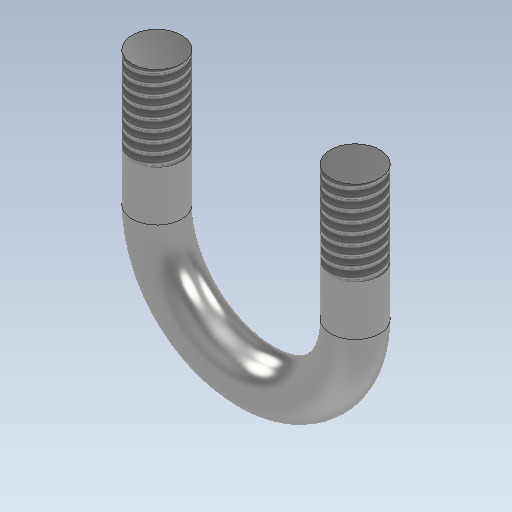
# Autodesk Inventor part: 19mm ID UBOLT
Saved by Autodesk Inventor 2023 (Build 270158000, 158)
## iProperties
Created: 2019-06-17
Part Number: 19mm ID UBOLT
Material: Stainless Steel, 440C
Document SubType Name: Modeling
Designer: pepd9
Density: 7.75 g/cm^3
Appearance: Semi-Polished
Description: FROG BEARING SUPPORTS
Author: pepd9
Autodesk Inventor part; units mm, degrees
ref_plane "YZ Plane" through (0, 0, 0) normal (1, 0, 0) x (0, 1, 0)
ref_plane "XZ Plane" through (0, 0, 0) normal (0, 1, 0) x (-1, 0, 0)
ref_plane "XY Plane" through (0, 0, 0) normal (0, 0, 1) x (1, 0, 0)
sketch "Sketch1" plane through (0, 0, 0) normal (0, 1, 0) x (-1, 0, 0)
  circle A0 centre (12.7, 0) radius 3.175
  line L0 (0, -4.445) -> (0, 4.445) projected
  point P0 (0, 0)
  dimension "d0" = 12.7
  dimension "d1" = 6.35
  constraints: 1 centre point
  measures "d0" distance of point (0, 0) A0.centre
  measures "d1" diameter of A0
revolve "Revolution1" add sketch "Sketch1" angle 180 about axis through (0, 0, -10) along (0, 0, 1)
sketch "Sketch2" plane through (-12.7, 0, 0) normal (0, 1, 0) x (1, 0, 0)
  circle A0 centre (0, 0) radius 3.175 projected
  circle A1 centre (25.4, 0) radius 3.175 projected
  point P0 (12.7, 0)
extrude "Extrusion1" add sketch "Sketch2" along normal blind 6.35
sketch "Sketch3" plane through (-12.7, 6.35, 0) normal (0, 1, 0) x (1, 0, 0)
  circle A0 centre (0, 0) radius 3.175 projected
  circle A1 centre (25.4, 0) radius 3.175 projected
  point P0 (12.7, 0)
extrude "Extrusion2" add sketch "Sketch3" along normal blind 15.875
thread "Thread1" size "1/4-20 UNC" class "2A" standard "ANSI Unified Screw Threads" length 15.875
thread "Thread2" size "1/4-20 UNC" class "2A" standard "ANSI Unified Screw Threads" length 15.875
sketch "Sketch4" plane through (-12.7, 22.225, 0) normal (0, 1, 0) x (1, 0, 0)
  line L0 (-3.2033, 0) -> (28.6033, 0) construction
  line L1 (-3.2033, -3.175) -> (28.6033, -3.175)
  line L2 (28.6033, 3.175) -> (-3.2033, 3.175)
  arc A0 (-3.2033, 3.175) -> (-3.2033, -3.175) centre (-3.2033, 0) ccw
  arc A1 (28.6033, -3.175) -> (28.6033, 3.175) centre (28.6033, 0) ccw
  point P0 (12.7, 0)
  constraints: 8 end point, 4 point on circle, 4 tangent, 2 centre point, 1 horizontal, 1 midpoint, 1 parallel
extrude "Extrusion3" cut sketch "Sketch4" against normal blind 5
body "Solid1"
